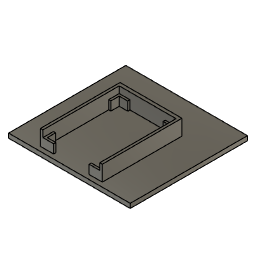
Mini PC - Bottom Plate (Autodesk Fusion 360 design; units mm, degrees)
Autodesk Fusion 360 part; units mm, degrees
sketch "Skizze1" plane through (0, 0, 0) normal (0, 0, 1) x (1, 0, 0)
  line L0 (-29.7708, 25.7681) -> (25.2292, 25.7681)
  line L1 (25.2292, 25.7681) -> (25.2292, -27.2319)
  line L2 (25.2292, -27.2319) -> (-29.7708, -27.2319)
  line L3 (-29.7708, -27.2319) -> (-29.7708, 25.7681)
  line L4 (9.4497, -27.2319) -> (-16.2503, -27.2319)
  line L5 (-16.2503, -27.2319) -> (-16.2503, 7.2681)
  line L6 (-16.2503, 7.2681) -> (9.4497, 7.2681)
  line L7 (9.4497, 7.2681) -> (9.4497, -27.2319)
  line L8 (9.4497, 2.5181) -> (8.4497, 2.5181)
  line L9 (8.4497, 2.5181) -> (8.4497, -22.4819)
  line L10 (8.4497, -22.4819) -> (9.4497, -22.4819)
  line L11 (9.4497, -22.4819) -> (9.4497, 2.5181)
  line L12 (-16.2503, 2.5181) -> (-15.2503, 2.5181)
  line L13 (-15.2503, 2.5181) -> (-15.2503, -22.4819)
  line L14 (-15.2503, -22.4819) -> (-16.2503, -22.4819)
  line L15 (-16.2503, -22.4819) -> (-16.2503, 2.5181)
  line L16 (-11.4003, 7.2681) -> (4.5997, 7.2681)
  line L17 (4.5997, 7.2681) -> (4.5997, 6.2681)
  line L18 (4.5997, 6.2681) -> (-11.4003, 6.2681)
  line L19 (-11.4003, 6.2681) -> (-11.4003, 7.2681)
  line L20 (-11.4003, -27.2319) -> (4.5997, -27.2319)
  line L21 (4.5997, -27.2319) -> (4.5997, -26.2319)
  line L22 (4.5997, -26.2319) -> (-11.4003, -26.2319)
  line L23 (-11.4003, -26.2319) -> (-11.4003, -27.2319)
  line L24 (-15.2503, 6.2681) -> (8.4497, 6.2681)
  line L25 (8.4497, 6.2681) -> (8.4497, -26.2319)
  line L26 (8.4497, -26.2319) -> (-15.2503, -26.2319)
  line L27 (-15.2503, -26.2319) -> (-15.2503, 6.2681)
  line L28 (-17.4003, 8.7681) -> (10.5997, 8.7681)
  line L29 (10.5997, 8.7681) -> (10.5997, -27.2319)
  line L30 (10.5997, -27.2319) -> (-17.4003, -27.2319)
  line L31 (-17.4003, -27.2319) -> (-17.4003, 8.7681)
  line L32 (8.4497, -26.2319) -> (9.4497, -26.2319)
  point P0 (8.4497, -9.9819)
  point P1 (9.4497, -9.9819)
  point P2 (-15.2503, -9.9819)
  point P3 (-3.4003, -27.2319)
  point P4 (-3.4003, 6.2681)
  point P5 (-3.4003, -26.2319)
  point P6 (-3.4003, 6.2681)
  point P7 (-3.4003, 8.7681)
  dimension "d5" = 55
  dimension "d6" = 53
  dimension "d7" = 34.5
  dimension "d8" = 25.7
  dimension "d9" = 25
  dimension "d10" = 1
  dimension "d11" = 1
  dimension "d12" = 16
  dimension "d13" = 32.5
  dimension "d14" = 23.7
  dimension "d17" = 28
  dimension "d18" = 36
  constraint horizontal L0
  constraint vertical L1
  constraint horizontal L2
  constraint vertical L3
  constraint horizontal L4
  constraint vertical L5
  constraint horizontal L6
  constraint vertical L7
  constraint coincident L2 L4.start
  constraint horizontal L8
  constraint vertical L9
  constraint horizontal L10
  constraint vertical L11
  constraint coincident L7 L8.start
  constraint midpoint L9 P0
  constraint midpoint L7 P1
  constraint horizontal P0 P1
  constraint horizontal L12
  constraint vertical L13
  constraint horizontal L14
  constraint vertical L15
  constraint coincident L5 L12.start
  constraint equal L9 L13
  constraint midpoint L13 P2
  constraint horizontal P1 P2
  constraint horizontal L16
  constraint vertical L17
  constraint horizontal L18
  constraint vertical L19
  constraint coincident L6 L16.start
  constraint equal L10 L19
  constraint midpoint L4 P3
  constraint midpoint L18 P6
  constraint vertical P3 P6
  constraint horizontal L20
  constraint vertical L21
  constraint horizontal L22
  constraint vertical L23
  constraint coincident L4 L20.start
  constraint equal L18 L22
  constraint equal L8 L21
  constraint midpoint L22 P5
  constraint vertical P3 P5
  constraint horizontal L24
  constraint vertical L25
  constraint horizontal L26
  constraint vertical L27
  constraint midpoint L24 P6
  constraint horizontal L28
  constraint vertical L29
  constraint horizontal L30
  constraint vertical L31
  constraint coincident L2 L29.end
  constraint midpoint L28 P7
  constraint vertical P6 P7
  constraint coincident L7 L32.end
  constraint perpendicular L7 L32
  measures "d5" distance of L0.start L0.end
  measures "d6" distance of L0.start L2.end
  measures "d7" distance of L4.start L6.end
  measures "d8" distance of L5.end L6.end
  measures "d9" distance of L8.end L9.end
  measures "d10" distance of L8.start L8.end
  measures "d11" distance of L12.start L12.end
  measures "d12" distance of L16.start L16.end
  measures "d13" distance of L24.end L25.end
  measures "d14" distance of L24.start L24.end
  measures "d17" distance of L28.start L28.end
  measures "d18" distance of L28.start L30.end
extrude "Extrusion1" add sketch "Skizze1" along normal blind 2 makes body 1
extrude "Extrusion2" add sketch "Skizze1" along normal blind 10 separate body contours L2 L5 L6 L7 L11 L15 L16 L28 L29 L30 L31 makes body 2
extrude "Extrusion3" add sketch "Skizze1" along normal blind 8 contours L2 L4 L5 L14 L23 L26 L27 L30 | L5 L6 L12 L19 L24 L27 | L6 L7 L8 L17 L24 L25 bodies 2
extrude "Extrusion4" cut 3 faces at (7.4997, 6.9348, 8) (-14.3003, 6.9348, 8) (-14.3003, -26.8986, 8) along direction (0, 0, -1) blind 4 on bodies 2 bodies 2
extrude "Extrusion5" cut 1 faces at (-7.6836, 8.2681, 10) along direction (0, 0, -1) blind 4 on bodies 2 bodies 2
extrude "Extrusion6" add 3 faces at (7.4997, 6.9348, 4) (-14.3003, 6.9348, 4) (-14.3003, -26.8986, 4) along direction (0, 0, 1) blind 1 on bodies 2 bodies 2
extrude "Extrusion7" add 1 faces at (-7.6836, 8.2681, 6) along direction (0, 0, 1) blind 1 on bodies 2 bodies 2
move_body "Verschieben1" bodies 1 to x (1, 0, 0) y (0, 1, 0) z (0, 0, 1) at (0, 0, -2)
extrude "Extrusion8" cut 3 faces at (7.4997, 6.9348, 5) (-14.3003, 6.9348, 5) (-14.3003, -26.8986, 5) along direction (0, 0, -1) blind 2 on bodies 2 bodies 2
extrude "Extrusion9" cut 1 faces at (-7.6836, 8.2681, 7) along direction (0, 0, -1) blind 2 on bodies 2 bodies 2
extrude "Extrusion10" cut 1 faces at (-11.4375, 25.7681, -1.3333) along direction (0, -1, 0) blind 2 on bodies 1 bodies 1
extrude "Extrusion11" add 1 faces at (6.8958, -27.2319, -0.6667) along direction (0, -1, 0) blind 2 on bodies 1 bodies 1 2
extrude "Extrusion12" add 1 faces at (-7.6836, 8.2681, 5) along direction (0, 0, 1) blind 2 on bodies 1 bodies 1
extrude "Extrusion13" add 3 faces at (7.4997, 6.9348, 3) (-14.3003, 6.9348, 3) (-14.3003, -26.8986, 3) along direction (0, 0, 1) blind 2 on bodies 1 bodies 1
extrude "Extrusion14" cut 3 faces at (7.4997, 6.9348, 5) (-14.3003, 6.9348, 5) (-14.3003, -26.8986, 5) along direction (0, 0, -1) blind 1 on bodies 1 bodies 1
extrude "Extrusion15" add sketch "Skizze1" along normal blind 4 contours L2 L4 L7 L21 L26 L30 L32 bodies 1
